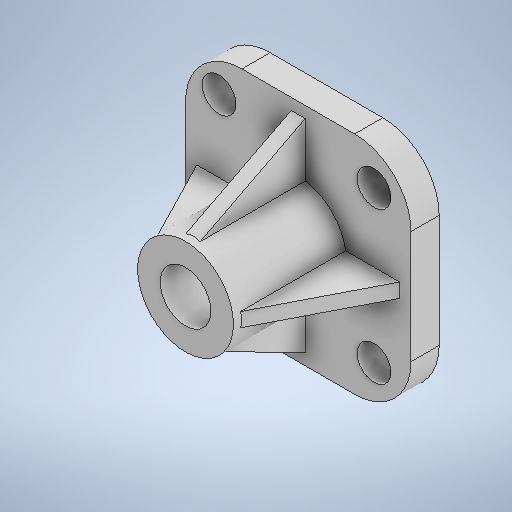
# Autodesk Inventor part: cad@62
Saved by Autodesk Inventor 2025.2 (Build 292293000, 293)
## iProperties
Created: 2025-04-21
Part Number: cad@62
Material: Generic
Document SubType Name: Modeling
Designer: spars
Density: 1 g/cm^3
Appearance: Default
Author: spars
Autodesk Inventor part; units mm, degrees
ref_plane "YZ Plane" through (0, 0, 0) normal (1, 0, 0) x (0, 1, 0)
ref_plane "XZ Plane" through (0, 0, 0) normal (0, 1, 0) x (-1, 0, 0)
ref_plane "XY Plane" through (0, 0, 0) normal (0, 0, 1) x (1, 0, 0)
sketch "Sketch1" plane through (0, 0, 0) normal (0, 0, 1) x (1, 0, 0)
  line L0 (-370.6622, 75.5496) -> (-164.0576, 75.5496) construction
  line L1 (-164.0576, 75.5496) -> (-164.0576, -88.718) construction
  line L2 (-164.0576, -88.718) -> (-370.6622, -88.718) construction
  line L3 (-370.6622, -88.718) -> (-370.6622, 75.5496) construction
  line L4 (-20, 40) -> (20, 40)
  line L5 (40, 20) -> (40, -20)
  line L6 (20, -40) -> (-20, -40)
  line L7 (-40, -20) -> (-40, 20)
  line L8 (-40, 40) -> (40, -40) construction
  line L9 (40, 40) -> (-40, -40) construction
  arc A0 (-20, 40) -> (-40, 20) centre (-20, 20) ccw
  arc A1 (-40, -20) -> (-20, -40) centre (-20, -20) ccw
  arc A2 (40, 20) -> (20, 40) centre (20, 20) ccw
  arc A3 (20, -40) -> (40, -20) centre (20, -20) ccw
  circle A4 centre (26.8834, -26.8834) radius 6
  circle A5 centre (-28.1031, -28.1031) radius 6
  circle A6 centre (26.8834, 26.8834) radius 6
  circle A7 centre (-28.1031, 28.1031) radius 6
  point P0 (0, 0)
  dimension "d5" = 80
  dimension "d6" = 80
  dimension "d7" = 20
  dimension "d9" = 12
  dimension "d11" = 12
  dimension "d12" = 55
  constraints: 12 end point, 10 point on line, 8 centre point, 8 point on circle, 8 tangent, 3 equal radius, 2 midpoint, 2 parallel, 1 horizontal, 1 perpendicular, 2 other
  measures "d5" distance of L8.end L9.end
  measures "d6" distance of L9.start L8.end
  measures "d7" radius of A0
  measures "d9" diameter of A4
  measures "d11" diameter of A5
  measures "d12" distance of A4.centre A5.centre
extrude "Extrusion1" add sketch "Sketch1" along normal blind 10
sketch "Sketch2" plane through (0, 0, 10) normal (0, 0, 1) x (1, 0, 0)
  circle A0 centre (0, 0) radius 17
  circle A1 centre (0, 0) radius 9
  dimension "d16" = 34
  dimension "d17" = 18
  constraints: 2 centre point, 2 coincident
  measures "d16" diameter of A0
  measures "d17" diameter of A1
extrude "Extrusion2" add sketch "Sketch2" along normal blind 40
sketch "Sketch3" plane through (0, 0, 0) normal (1, 0, 0) x (0, 1, 0)
  point P0 (0, 0)
sketch "Sketch4" plane through (0, 0, 0) normal (1, 0, 0) x (0, 1, 0)
  line L0 (-20.9926, 39.225) -> (-30, 21.6842)
  point P0 (0, 0)
  point P1 (-40, 10)
  constraints: 2 end point
extrude "Rib1" add sketch "Sketch4" along normal mid plane 5 rib yes fills toward (-25.4518, 30.4318) open curves L0
pattern_circular "Circular Pattern1" count 4 over 360 about axis through (0, 0, 10) along (0, 0, 1) of "Rib1"
body "Solid1"
